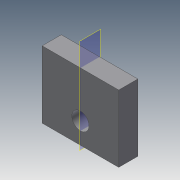
# Autodesk Inventor part: Y screw bracket
Saved by Autodesk Inventor 2019 (Build 230136000, 136)
## iProperties
Created: 2019-02-27
Part Number: Y screw bracket
Material: Generic
Document SubType Name: Modeling
Designer: LillaHunden
Density: 1 g/cm^3
Appearance: Default
Author: LillaHunden
Autodesk Inventor part; units mm, degrees
ref_plane "YZ Plane" through (0, 0, 0) normal (1, 0, 0) x (0, 1, 0)
ref_plane "XZ Plane" through (0, 0, 0) normal (0, 1, 0) x (-1, 0, 0)
ref_plane "XY Plane" through (0, 0, 0) normal (0, 0, 1) x (1, 0, 0)
sketch "Sketch1" plane through (0, 0, 0) normal (0, 0, 1) x (1, 0, 0)
  line L0 (-30.1791, 10) -> (-70.1791, 10)
  line L1 (-70.1791, 10) -> (-70.1791, 45)
  line L2 (-70.1791, 45) -> (-30.1791, 45)
  line L3 (-30.1791, 45) -> (-30.1791, 10)
  point P0 (0, 0)
  dimension "d0" = 40
  dimension "d1" = 35
  constraints: 8 end point, 2 parallel, 1 horizontal, 1 perpendicular
  measures "d0" distance of L1.end L2.end
  measures "d1" distance of L0.end L1.end
extrude "Extrusion1" add sketch "Sketch1" along normal blind 10
ref_plane "Work Plane1" through (-50.1791, 10, 0) normal (-1, 0, 0) x (0, 0, 1)
sketch "Sketch2" plane through (0, 0, 0) normal (0, 0, -1) x (-1, 0, 0)
  circle A0 centre (50.1791, 21) radius 4.5 projected
  point P0 (0, 0)
extrude "Extrusion2" cut sketch "Sketch2" against normal through all
sketch "Sketch3" plane through (0, 0, 0) normal (0, 0, -1) x (-1, 0, 0)
  circle A0 centre (50.1791, 21) radius 11 construction
  spline S0 degree 3 poles (41.3737, 19.4605) (41.4379, 19.6108) (41.5322, 19.7457) (41.6483, 19.8612) (41.6554, 19.8683) (41.6627, 19.8753) (41.67, 19.8823) (41.7783, 19.9853) (41.9027, 20.0701) (42.0377, 20.1333) (42.0529, 20.1405) (42.0683, 20.1473) (42.0838, 20.1539) (42.0941, 20.1583) (42.1044, 20.1625) (42.1147, 20.1666) (42.1989, 20.1998) (42.2859, 20.2245) (42.3745, 20.2398) (42.4286, 20.2491) (42.4834, 20.2549) (42.5385, 20.2574) (42.555, 20.2581) (42.5716, 20.2586) (42.5881, 20.2587) (42.6034, 20.2589) (42.6187, 20.2587) (42.6341, 20.2584) (42.7841, 20.2547) (42.9332, 20.2271) (43.0761, 20.1784) (43.0946, 20.1721) (43.113, 20.1654) (43.1313, 20.1584) (43.1423, 20.1542) (43.1532, 20.1499) (43.1642, 20.1454) (43.2564, 20.1076) (43.3448, 20.061) (43.4277, 20.0063) (43.4412, 19.9974) (43.4545, 19.9883) (43.4677, 19.979) (43.4774, 19.9721) (43.487, 19.9652) (43.4965, 19.9581) (43.5453, 19.9219) (43.5918, 19.8827) (43.6356, 19.8408) (43.6561, 19.8212) (43.676, 19.8009) (43.6953, 19.7801) (43.7118, 19.7622) (43.7279, 19.7439) (43.7417, 19.7234) knots 0 0 0 0 0.171917 0.171917 0.171917 0.182531 0.182531 0.182531 0.339556 0.339556 0.339556 0.35729 0.35729 0.35729 0.369023 0.369023 0.369023 0.464442 0.464442 0.464442 0.522742 0.522742 0.522742 0.540193 0.540193 0.540193 0.556325 0.556325 0.556325 0.714368 0.714368 0.714368 0.734813 0.734813 0.734813 0.747126 0.747126 0.747126 0.851246 0.851246 0.851246 0.868176 0.868176 0.868176 0.880588 0.880588 0.880588 0.944403 0.944403 0.944403 0.974326 0.974326 0.974326 1 1 1 1 construction
  arc A1 (43.4969, 17.684) -> (43.7415, 19.7236) centre (42.476, 18.8409) ccw construction
  spline S1 degree 3 poles (43.4969, 17.684) (43.3425, 17.5704) (43.1671, 17.4889) (42.9813, 17.4411) (42.9692, 17.438) (42.9569, 17.435) (42.9447, 17.4322) (42.7683, 17.3914) (42.5862, 17.3816) (42.4079, 17.4054) (42.3978, 17.4068) (42.3878, 17.4082) (42.3778, 17.4098) (42.2858, 17.4241) (42.1959, 17.4475) (42.1093, 17.4803) (42.058, 17.4998) (42.0078, 17.5225) (41.959, 17.5484) (41.9439, 17.5564) (41.929, 17.5647) (41.9142, 17.5733) (41.9013, 17.5809) (41.8884, 17.5886) (41.8756, 17.5966) (41.7356, 17.6842) (41.6116, 17.7967) (41.5102, 17.9279) (41.5034, 17.9367) (41.4967, 17.9455) (41.4901, 17.9545) (41.4384, 18.0248) (41.3935, 18.0997) (41.3566, 18.1783) (41.3513, 18.1894) (41.3463, 18.2005) (41.3414, 18.2118) (41.3094, 18.2853) (41.2845, 18.3614) (41.2676, 18.4395) (41.2634, 18.4591) (41.2597, 18.4789) (41.2584, 18.4996) knots 0 0 0 0 0.200829 0.200829 0.200829 0.213978 0.213978 0.213978 0.403633 0.403633 0.403633 0.414319 0.414319 0.414319 0.512539 0.512539 0.512539 0.570815 0.570815 0.570815 0.588808 0.588808 0.588808 0.60461 0.60461 0.60461 0.77833 0.77833 0.77833 0.789949 0.789949 0.789949 0.881423 0.881423 0.881423 0.894318 0.894318 0.894318 0.978751 0.978751 0.978751 1 1 1 1 construction
  arc A2 (41.3737, 19.4605) -> (41.2584, 18.4996) centre (42.476, 18.8409) ccw construction
  spline S2 degree 3 poles (51.2359, 13.9165) (51.2931, 14.0503) (51.3742, 14.1719) (51.4731, 14.2785) (51.4853, 14.2916) (51.4978, 14.3045) (51.5105, 14.3171) (51.5177, 14.3243) (51.5249, 14.3313) (51.5323, 14.3383) (51.6406, 14.4413) (51.765, 14.5261) (51.8999, 14.5893) (51.9152, 14.5965) (51.9306, 14.6033) (51.9461, 14.6099) (51.9563, 14.6142) (51.9666, 14.6185) (51.977, 14.6226) (52.0612, 14.6558) (52.1481, 14.6805) (52.2367, 14.6957) (52.2909, 14.7051) (52.3457, 14.7109) (52.4008, 14.7134) (52.4173, 14.7141) (52.4338, 14.7146) (52.4504, 14.7147) (52.4657, 14.7149) (52.481, 14.7147) (52.4963, 14.7144) (52.6658, 14.7102) (52.8341, 14.6756) (52.9935, 14.6144) (53.0045, 14.6102) (53.0155, 14.6059) (53.0264, 14.6014) (53.1187, 14.5636) (53.207, 14.517) (53.29, 14.4623) (53.3034, 14.4534) (53.3168, 14.4443) (53.33, 14.435) (53.3397, 14.4281) (53.3492, 14.4212) (53.3587, 14.4141) (53.4305, 14.3608) (53.4971, 14.3014) (53.5575, 14.2361) (53.5741, 14.2182) (53.5902, 14.1999) (53.6039, 14.1794) knots 0 0 0 0 0.153066 0.153066 0.153066 0.171917 0.171917 0.171917 0.182531 0.182531 0.182531 0.339556 0.339556 0.339556 0.35729 0.35729 0.35729 0.369023 0.369023 0.369023 0.464442 0.464442 0.464442 0.522742 0.522742 0.522742 0.540193 0.540193 0.540193 0.556325 0.556325 0.556325 0.734813 0.734813 0.734813 0.747126 0.747126 0.747126 0.851246 0.851246 0.851246 0.868176 0.868176 0.868176 0.880588 0.880588 0.880588 0.974326 0.974326 0.974326 1 1 1 1 construction
  arc A3 (53.3592, 12.1399) -> (53.6038, 14.1796) centre (52.3382, 13.2969) ccw construction
  spline S3 degree 3 poles (53.3592, 12.1399) (53.2239, 12.0405) (53.0726, 11.9657) (52.9124, 11.9165) (52.8896, 11.9095) (52.8667, 11.9031) (52.8436, 11.8971) (52.8314, 11.894) (52.8192, 11.891) (52.807, 11.8882) (52.6519, 11.8523) (52.4925, 11.8404) (52.3351, 11.8542) (52.3134, 11.8561) (52.2918, 11.8585) (52.2701, 11.8614) (52.2601, 11.8628) (52.2501, 11.8642) (52.2401, 11.8658) (52.1481, 11.8801) (52.0582, 11.9035) (51.9716, 11.9363) (51.9202, 11.9557) (51.87, 11.9785) (51.8213, 12.0044) (51.8062, 12.0124) (51.7913, 12.0207) (51.7765, 12.0293) (51.7635, 12.0368) (51.7506, 12.0446) (51.7379, 12.0526) (51.6134, 12.1305) (51.5016, 12.2281) (51.407, 12.3409) (51.3952, 12.355) (51.3837, 12.3693) (51.3724, 12.3839) (51.3656, 12.3927) (51.3589, 12.4015) (51.3524, 12.4105) (51.3006, 12.4808) (51.2558, 12.5557) (51.2188, 12.6343) (51.2136, 12.6454) (51.2085, 12.6565) (51.2037, 12.6678) (51.1717, 12.7412) (51.1467, 12.8174) (51.1299, 12.8955) (51.1256, 12.9151) (51.1219, 12.9349) (51.1206, 12.9556) knots 0 0 0 0 0.175859 0.175859 0.175859 0.200829 0.200829 0.200829 0.213978 0.213978 0.213978 0.380655 0.380655 0.380655 0.403633 0.403633 0.403633 0.414319 0.414319 0.414319 0.512539 0.512539 0.512539 0.570815 0.570815 0.570815 0.588808 0.588808 0.588808 0.60461 0.60461 0.60461 0.759068 0.759068 0.759068 0.77833 0.77833 0.77833 0.789949 0.789949 0.789949 0.881423 0.881423 0.881423 0.894318 0.894318 0.894318 0.978751 0.978751 0.978751 1 1 1 1 construction
  arc A4 (51.2359, 13.9165) -> (51.1206, 12.9556) centre (52.3382, 13.2969) ccw construction
  spline S4 degree 3 poles (56.78, 23.7788) (56.8441, 23.929) (56.9384, 24.064) (57.0545, 24.1794) (57.0617, 24.1865) (57.0689, 24.1936) (57.0763, 24.2005) (57.1846, 24.3036) (57.309, 24.3884) (57.4439, 24.4516) (57.4592, 24.4587) (57.4746, 24.4656) (57.4901, 24.4721) (57.5003, 24.4765) (57.5106, 24.4807) (57.521, 24.4848) (57.6052, 24.5181) (57.6921, 24.5427) (57.7808, 24.558) (57.8349, 24.5673) (57.8897, 24.5732) (57.9448, 24.5756) (57.9613, 24.5764) (57.9778, 24.5768) (57.9944, 24.577) (58.0097, 24.5771) (58.025, 24.577) (58.0403, 24.5766) (58.2098, 24.5724) (58.3781, 24.5378) (58.5375, 24.4767) (58.5485, 24.4725) (58.5595, 24.4681) (58.5704, 24.4636) (58.6627, 24.4258) (58.751, 24.3792) (58.834, 24.3245) (58.8475, 24.3156) (58.8608, 24.3065) (58.874, 24.2972) (58.8837, 24.2904) (58.8933, 24.2834) (58.9028, 24.2764) (58.9745, 24.2231) (59.0411, 24.1636) (59.1016, 24.0983) (59.1181, 24.0805) (59.1342, 24.0621) (59.1479, 24.0417) knots 0 0 0 0 0.171917 0.171917 0.171917 0.182531 0.182531 0.182531 0.339556 0.339556 0.339556 0.35729 0.35729 0.35729 0.369023 0.369023 0.369023 0.464442 0.464442 0.464442 0.522742 0.522742 0.522742 0.540193 0.540193 0.540193 0.556325 0.556325 0.556325 0.734813 0.734813 0.734813 0.747125 0.747125 0.747125 0.851246 0.851246 0.851246 0.868176 0.868176 0.868176 0.880588 0.880588 0.880588 0.974325 0.974325 0.974325 1 1 1 1 construction
  arc A5 (58.9032, 22.0022) -> (59.1478, 24.0418) centre (57.8822, 23.1591) ccw construction
  spline S5 degree 3 poles (58.9032, 22.0022) (58.768, 21.9028) (58.6166, 21.828) (58.4564, 21.7788) (58.4336, 21.7718) (58.4107, 21.7653) (58.3876, 21.7594) (58.3754, 21.7562) (58.3632, 21.7533) (58.351, 21.7504) (58.1745, 21.7096) (57.9925, 21.6998) (57.8142, 21.7237) (57.8041, 21.725) (57.7941, 21.7265) (57.7841, 21.728) (57.6921, 21.7424) (57.6022, 21.7657) (57.5156, 21.7985) (57.4484, 21.824) (57.3832, 21.8552) (57.3205, 21.8916) (57.3075, 21.8991) (57.2946, 21.9069) (57.2819, 21.9148) (57.1574, 21.9927) (57.0456, 22.0903) (56.951, 22.2032) (56.9392, 22.2173) (56.9277, 22.2316) (56.9164, 22.2461) (56.9096, 22.2549) (56.9029, 22.2638) (56.8964, 22.2727) (56.8447, 22.343) (56.7998, 22.4179) (56.7628, 22.4965) (56.7576, 22.5076) (56.7526, 22.5188) (56.7477, 22.53) (56.7157, 22.6035) (56.6908, 22.6796) (56.6739, 22.7577) (56.6697, 22.7774) (56.6659, 22.7971) (56.6646, 22.8179) knots 0 0 0 0 0.175859 0.175859 0.175859 0.200829 0.200829 0.200829 0.213978 0.213978 0.213978 0.403633 0.403633 0.403633 0.414319 0.414319 0.414319 0.512539 0.512539 0.512539 0.588808 0.588808 0.588808 0.60461 0.60461 0.60461 0.759068 0.759068 0.759068 0.77833 0.77833 0.77833 0.789949 0.789949 0.789949 0.881423 0.881423 0.881423 0.894318 0.894318 0.894318 0.978751 0.978751 0.978751 1 1 1 1 construction
  arc A6 (56.78, 23.7788) -> (56.6646, 22.8179) centre (57.8822, 23.1591) ccw construction
  spline S6 degree 3 poles (46.9177, 29.3228) (46.9748, 29.4566) (47.0559, 29.5782) (47.1549, 29.6847) (47.1671, 29.6979) (47.1795, 29.7107) (47.1923, 29.7234) (47.1994, 29.7305) (47.2067, 29.7376) (47.214, 29.7445) (47.3224, 29.8476) (47.4467, 29.9324) (47.5817, 29.9956) (47.5969, 30.0027) (47.6123, 30.0096) (47.6278, 30.0161) (47.6381, 30.0205) (47.6484, 30.0247) (47.6588, 30.0288) (47.7429, 30.0621) (47.8299, 30.0867) (47.9185, 30.102) (47.9727, 30.1113) (48.0274, 30.1172) (48.0825, 30.1197) (48.099, 30.1204) (48.1156, 30.1208) (48.1321, 30.121) (48.1474, 30.1211) (48.1628, 30.121) (48.1781, 30.1206) (48.3475, 30.1165) (48.5158, 30.0819) (48.6753, 30.0207) (48.6863, 30.0165) (48.6973, 30.0121) (48.7082, 30.0076) (48.8154, 29.9637) (48.9174, 29.9079) (49.0117, 29.8412) (49.0945, 29.7828) (49.1709, 29.7163) (49.2393, 29.6423) (49.2559, 29.6245) (49.2719, 29.6062) (49.2857, 29.5857) knots 0 0 0 0 0.153066 0.153066 0.153066 0.171917 0.171917 0.171917 0.182531 0.182531 0.182531 0.339556 0.339556 0.339556 0.35729 0.35729 0.35729 0.369023 0.369023 0.369023 0.464442 0.464442 0.464442 0.522742 0.522742 0.522742 0.540193 0.540193 0.540193 0.556325 0.556325 0.556325 0.734813 0.734813 0.734813 0.747125 0.747125 0.747125 0.868176 0.868176 0.868176 0.974325 0.974325 0.974325 1 1 1 1 construction
  arc A7 (49.0409, 27.5462) -> (49.2856, 29.5858) centre (48.02, 28.7031) ccw construction
  spline S7 degree 3 poles (49.0409, 27.5462) (48.8865, 27.4327) (48.7111, 27.3511) (48.5253, 27.3034) (48.5132, 27.3002) (48.501, 27.2973) (48.4887, 27.2944) (48.3337, 27.2586) (48.1743, 27.2467) (48.0169, 27.2605) (47.9952, 27.2624) (47.9735, 27.2648) (47.9519, 27.2677) (47.9419, 27.269) (47.9318, 27.2705) (47.9218, 27.272) (47.8299, 27.2864) (47.7399, 27.3098) (47.6533, 27.3425) (47.602, 27.362) (47.5518, 27.3848) (47.503, 27.4107) (47.488, 27.4187) (47.473, 27.427) (47.4583, 27.4356) (47.4453, 27.4431) (47.4324, 27.4509) (47.4197, 27.4588) (47.2951, 27.5368) (47.1834, 27.6343) (47.0887, 27.7472) (47.0769, 27.7613) (47.0654, 27.7756) (47.0542, 27.7902) (47.0474, 27.7989) (47.0407, 27.8078) (47.0341, 27.8167) (46.9824, 27.887) (46.9375, 27.9619) (46.9006, 28.0405) (46.8954, 28.0516) (46.8903, 28.0628) (46.8854, 28.074) (46.8534, 28.1475) (46.8285, 28.2236) (46.8117, 28.3017) (46.8074, 28.3214) (46.8037, 28.3411) (46.8024, 28.3619) knots 0 0 0 0 0.200829 0.200829 0.200829 0.213978 0.213978 0.213978 0.380655 0.380655 0.380655 0.403633 0.403633 0.403633 0.414319 0.414319 0.414319 0.512539 0.512539 0.512539 0.570815 0.570815 0.570815 0.588808 0.588808 0.588808 0.60461 0.60461 0.60461 0.759068 0.759068 0.759068 0.77833 0.77833 0.77833 0.789949 0.789949 0.789949 0.881423 0.881423 0.881423 0.894318 0.894318 0.894318 0.978751 0.978751 0.978751 1 1 1 1 construction
  arc A8 (46.9177, 29.3228) -> (46.8024, 28.3619) centre (48.02, 28.7031) ccw construction
  circle A9 centre (50.1791, 21) radius 4.5 construction
  point P0 (0, 0)
hole "Hole1" at (-57.8822, 23.1591, 0) at (-48.02, 28.7031, 0) at (-42.476, 18.8409, 0) at (-52.3382, 13.2969, 0) direction (0, 0, 1) diameter 3.4 depth 8.8 clearance for "Socket Head Cap Screw ISO 4762" size "M3" standard "ISO"
sketch "Sketch4" plane through (-70.1791, 45, 0) normal (0, 1, 0) x (1, 0, 0)
  line L0 (0, 0) -> (0, -10) construction
  line L1 (0, -5) -> (40, -5) construction
  line L2 (40, 0) -> (40, -10) construction
  point P0 (70.1791, 0)
  point P1 (10, -5)
  point P2 (20, -5)
  point P3 (30, -5)
  dimension "d13" = 10
  dimension "d14" = 10
  dimension "d15" = 10
  constraints: 3 midpoint, 2 end point, 2 point on line
  measures "d13" distance from line of L0 point (10, -5)
  measures "d14" distance of point (20, -5) point (10, -5)
  measures "d15" distance of point (30, -5) point (20, -5)
sketch "Sketch5" plane through (-70.1791, 45, 0) normal (0, 1, 0) x (1, 0, 0)
  point P0 (10, -5)
  point P1 (20, -5)
  point P2 (30, -5)
hole "Hole2" at (-60.1791, 45, 5) at (-50.1791, 45, 5) at (-40.1791, 45, 5) direction (0, -1, 0) diameter 3.242 depth 10 tip angle 120 thread size "M4x0.7" class "6H" standard "ISO Metric profile"
equation "\"d14\" = d13"
equation "\"d15\" = d14"
body "Solid1"
